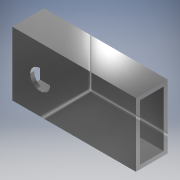
# Autodesk Inventor part: 15102898-16-P-0304
Saved by Autodesk Inventor 2017 (Build 210142000, 142)
## iProperties
Created: 2016-10-03
Part Number: 15102898-16-P-0304
Material: Aluminum 6061
Document SubType Name: Modeling
Designer: gus
Density: 2.7 g/cm^3
Appearance: Aluminum - Flat
Mass: 114.48 g
Surface Area: 280.39 cm^2
Volume: 42.3999 cm^3
Author: gus
Autodesk Inventor part; units mm, degrees
ref_plane "YZ Plane" through (0, 0, 0) normal (1, 0, 0) x (0, 1, 0)
ref_plane "XZ Plane" through (0, 0, 0) normal (0, 1, 0) x (-1, 0, 0)
ref_plane "XY Plane" through (0, 0, 0) normal (0, 0, 1) x (1, 0, 0)
sketch "Sketch1" plane through (0, 0, 0) normal (1, 0, 0) x (0, 1, 0)
  line L0 (0, 0) -> (50.8, 0)
  line L1 (50.8, 0) -> (50.8, -25.4)
  line L2 (50.8, -25.4) -> (0, -25.4)
  line L3 (0, -25.4) -> (0, 0)
  line L4 (47.625, -3.175) -> (3.175, -3.175)
  line L5 (3.175, -3.175) -> (3.175, -22.225)
  line L6 (3.175, -22.225) -> (47.625, -22.225)
  line L7 (47.625, -22.225) -> (47.625, -3.175)
  dimension "d0" = 50.8
  dimension "d1" = 25.4
  dimension "d2" = 3.175
  constraints: 16 end point, 4 parallel, 2 perpendicular, 1 horizontal, 3 other
  measures "d0" distance of L1.end L2.end
  measures "d1" distance of L0.end L1.end
  measures "d2" distance between parallel lines of L0 L4
extrude "Extrusion1" add sketch "Sketch1" along normal blind 98.425
sketch "Sketch2" plane through (0, 0, -25.4) normal (0, 0, -1) x (-1, 0, 0)
  line L0 (0, 50.8) -> (-98.425, 50.8) projected
  line L1 (0, 50.8) -> (0, 0) projected
  line L2 (0, 0) -> (-98.425, 0) projected
  point P0 (-22.225, 25.4)
  dimension "d5" = 25.4
  dimension "d6" = 22.225
  measures "d5" distance from line of L0 point (-22.225, 25.4)
  measures "d6" distance from line of L1 point (-22.225, 25.4)
hole "Hole1" at (22.225, 25.4, -25.4) direction (0, 0, 1) diameter 28.575 depth 3.175 tip angle 118
hole "Hole2" at (22.225, 25.4, -25.4) direction (0, 0, 1) diameter 15.875 end through all
sketch "Sketch3" plane through (0, 0, -25.4) normal (0, 0, -1) x (-1, 0, 0)
  circle A0 centre (-85.725, 12.7) radius 3.175
  circle A1 centre (-60.325, 41.275) radius 3.175
  line L0 (0, 0) -> (-98.425, 0) projected
  line L1 (-98.425, 0) -> (-98.425, 50.8) projected
  dimension "d23" = 6.35
  dimension "d24" = 6.35
  dimension "d25" = 12.7
  dimension "d26" = 38.1
  dimension "d27" = 41.275
  dimension "d28" = 12.7
  constraints: 2 centre point
  measures "d23" diameter of A0
  measures "d24" diameter of A1
  measures "d25" distance from line of L0 A0.centre
  measures "d26" distance from line of L1 A1.centre
  measures "d27" distance from line of L0 A1.centre
  measures "d28" distance from line of L1 A0.centre
extrude "Extrusion2" cut sketch "Sketch3" against normal blind 25.4
body "Solid1"
